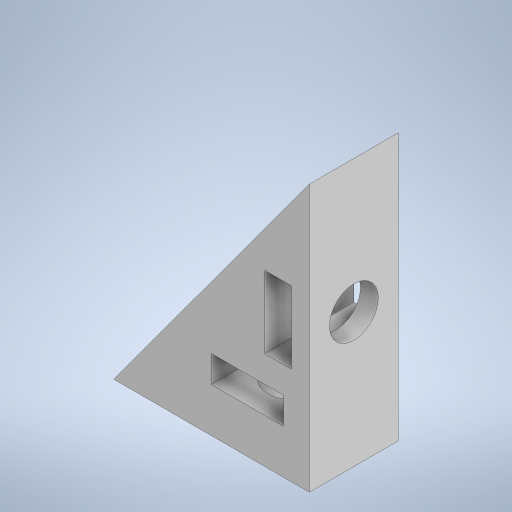
# Autodesk Inventor part: ligamento_obj4
Saved by Autodesk Inventor 2023.2 (Build 272271030, 271C)
## iProperties
Created: 2023-02-25
Part Number: ligamento_obj4
Material: Generic
Document SubType Name: Modeling
Designer: Cris Pat
Density: 1 g/cm^3
Appearance: Default
Author: Cris Pat
Autodesk Inventor part; units mm, degrees
ref_plane "YZ Plane" through (0, 0, 0) normal (1, 0, 0) x (0, 1, 0)
ref_plane "XZ Plane" through (0, 0, 0) normal (0, 1, 0) x (-1, 0, 0)
ref_plane "XY Plane" through (0, 0, 0) normal (0, 0, 1) x (1, 0, 0)
sketch "Sketch1" plane through (0, 0, 0) normal (0, 0, 1) x (1, 0, 0)
  line L0 (-11, 0) -> (11, 0)
  line L1 (11, 0) -> (11, 30)
  line L2 (11, 30) -> (-11, 0)
  point P0 (0, 0)
  point P1 (0, 0)
  dimension "d0" = 22
  dimension "d1" = 30
  constraints: 6 end point, 2 coincident, 1 horizontal, 1 midpoint, 1 vertical
  measures "d0" distance of L0.start L0.end
  measures "d1" distance of L0.end L1.end
extrude "Extrusion1" add sketch "Sketch1" along normal mid plane 10
sketch "Sketch2" plane through (0, 0, 0) normal (0, 0, 1) x (1, 0, 0)
  line L0 (11, 30) -> (11, 0) construction
  line L1 (11, 0) -> (-11, 0) construction
  line L2 (-11, 0) -> (11, 30) construction
  line L3 (8.1, 8) -> (0, 8)
  line L4 (0, 8) -> (0, 5)
  line L5 (0, 5) -> (8.1, 5)
  line L6 (8.1, 5) -> (8.1, 8)
  line L7 (6, 11) -> (9, 11)
  line L8 (9, 11) -> (9, 19.1)
  line L9 (9, 19.1) -> (6, 19.1)
  line L10 (6, 19.1) -> (6, 11)
  point P0 (0, 0)
  point P1 (0, 6.5)
  point P2 (0, 0)
  point P3 (11, 15)
  dimension "d4" = 8.1
  dimension "d5" = 5
  dimension "d6" = 3
  dimension "d7" = 3
  dimension "d8" = 8.1
  dimension "d9" = 2
  dimension "d10" = 3
  constraints: 16 end point, 4 parallel, 3 midpoint, 2 horizontal, 2 perpendicular, 1 vertical alignment
  measures "d4" distance from line of L6 point (0, 6.5)
  measures "d5" distance between parallel lines of L5 L1
  measures "d6" distance between parallel lines of L5 L3
  measures "d7" distance between parallel lines of L8 L10
  measures "d8" distance between parallel lines of L7 L9
  measures "d9" distance from line of point (11, 15) L8
  measures "d10" distance between parallel lines of L7 L3
extrude "Extrusion2" cut sketch "Sketch2" along normal through all both and the other way through all
sketch "Sketch3" plane through (11, 0, 5) normal (1, 0, 0) x (0, 0, -1)
  line L0 (10, 19.1) -> (10, 11) construction
  line L1 (10, 19.1) -> (0, 19.1) construction
  line L2 (0, 11) -> (0, 19.1) construction
  line L3 (10, 11) -> (0, 11) construction
  line L4 (10, 19.1) -> (0, 19.1) construction
  line L5 (5, 19.1) -> (5, 11) construction
  line L6 (0, 15.05) -> (10, 15.05) construction
  line L7 (10, 19.1) -> (10, 11) construction
  circle A0 centre (5, 15.05) radius 2.75
  point P0 (5, 0)
  dimension "d13" = 5.5
  constraints: 6 midpoint, 4 end point, 2 coincident, 1 centre point, 1 perpendicular
  measures "d13" diameter of A0
extrude "Extrusion3" cut sketch "Sketch3" against normal up to surface (5 mm away)
sketch "Sketch4" plane through (-11, 0, 5) normal (0, -1, 0) x (1, 0, 0)
  line L0 (19.1, -10) -> (11, -10) construction
  line L1 (19.1, -10) -> (19.1, 0) construction
  line L2 (11, 0) -> (19.1, 0) construction
  line L3 (11, 0) -> (11, -10) construction
  line L4 (19.1, 0) -> (11, 0) construction
  line L5 (15.05, 0) -> (15.05, -10) construction
  line L6 (19.1, -10) -> (11, -10) construction
  line L7 (11, -5) -> (19.1, -5) construction
  circle A0 centre (15.05, -5) radius 2.75
  dimension "d16" = 5.5
  constraints: 4 end point, 4 midpoint, 1 centre point, 1 coincident
  measures "d16" diameter of A0
extrude "Extrusion4" cut sketch "Sketch4" against normal up to surface (8 mm away)
body "Solid1"
